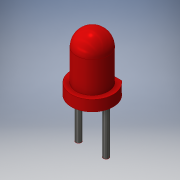
# Autodesk Inventor part: 3mm_LED
Saved by Autodesk Inventor 2016 (Build 200138000, 138)
## iProperties
Created: 2016-09-23
Part Number: 3mm_LED
Material: Generic
Document SubType Name: Modeling
Designer: jfixelle
Density: 1 g/cm^3
Appearance: Red
Author: jfixelle
Autodesk Inventor part; units mm, degrees
ref_plane "YZ Plane" through (0, 0, 0) normal (1, 0, 0) x (0, 1, 0)
ref_plane "XZ Plane" through (0, 0, 0) normal (0, 1, 0) x (-1, 0, 0)
ref_plane "XY Plane" through (0, 0, 0) normal (0, 0, 1) x (1, 0, 0)
sketch "Sketch1" plane through (0, 0, 0) normal (0, 1, 0) x (-1, 0, 0)
  arc A0 (1.2065, -1.5) -> (-1.2065, -1.5) centre (0, 0) ccw
  circle A1 centre (0, 0) radius 1.5
  line L0 (0, -1.5) -> (1.2065, -1.5)
  line L1 (0, -1.5) -> (-1.2065, -1.5)
  dimension "d1" = 3
  dimension "d0" = 3.85
  constraints: 4 end point, 2 coincident, 2 horizontal, 2 point on circle, 1 centre point, 1 point on line, 1 vertical alignment, 2 other
  measures "d0" diameter of A0
extrude "Extrusion1" add sketch "Sketch1" along normal blind 1 contours A1 | L0 L1 A0
sketch "Sketch2" plane through (0, 1, 0) normal (0, 1, 0) x (1, 0, 0)
  arc A0 (-1.2065, 1.5) -> (1.2065, 1.5) centre (0, 0) ccw projected
  circle A1 centre (0, 0) radius 1.47
  dimension "d4" = 2.94
  constraints: 1 centre point, 1 coincident
  measures "d4" diameter of A1
extrude "Extrusion2" add sketch "Sketch2" along normal blind 4.32
fillet "Fillet1" radius 1.47 1 edges at (-1.47, 5.32, 0)
sketch "Sketch3" plane through (0, 0, 0) normal (0, -1, 0) x (1, 0, 0)
  circle A0 centre (1.27, 0) radius 0.25
  circle A1 centre (-1.27, 0) radius 0.25
  point P0 (0, 0)
  dimension "d8" = 0.5
  dimension "d9" = 0.5
  dimension "d10" = 1.27
  dimension "d11" = 1.27
  constraints: 2 centre point
  measures "d8" diameter of A1
  measures "d9" diameter of A0
  measures "d10" distance of point (0, 0) A0.centre
  measures "d11" distance of A1.centre point (0, 0)
extrude "Extrusion3" add sketch "Sketch3" along normal blind 4.32
body "Solid1"
